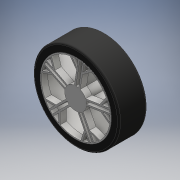
# Autodesk Inventor part: rueda
Saved by Autodesk Inventor 2016 (Build 200138000, 138)
## iProperties
Created: 2017-12-28
Part Number: rueda
Material: Genérico
Document SubType Name: Sheet Metal
Designer: David
Density: 1 g/cm^3
Sheet Metal Rule: Por defecto_mm
Appearance: Valor por defecto
Author: David
Autodesk Inventor part; units mm, degrees
ref_plane "YZ Plane" through (0, 0, 0) normal (1, 0, 0) x (0, 1, 0)
ref_plane "XZ Plane" through (0, 0, 0) normal (0, 1, 0) x (-1, 0, 0)
ref_plane "XY Plane" through (0, 0, 0) normal (0, 0, 1) x (1, 0, 0)
sketch "Boceto1" plane through (0, 0, 0) normal (0, 1, 0) x (-1, 0, 0)
  line L0 (0, 0) -> (10.7734, 0) construction
  line L1 (0, 0) -> (5.8764, 0) construction
  line L2 (0, 0) -> (5.8764, 0) construction
  line L3 (2.6962, -2.1086) -> (2.8923, -2.3046)
  line L4 (2.0927, -2.7086) -> (2.3729, -2.9905)
  line L5 (2.3729, -2.9905) -> (7.2915, -7.9381)
  line L6 (1.6666, -2.9897) -> (4.8298, -6.1715)
  line L7 (4.8298, -6.1715) -> (4.8298, -9.636)
  line L8 (5.3412, -9.3623) -> (5.3412, -6.6658)
  line L9 (5.3412, -6.6658) -> (6.9255, -8.2594)
  line L10 (2.6945, -2.1068) -> (2.9764, -2.387)
  line L11 (2.9764, -2.387) -> (7.924, -7.3056)
  line L12 (2.9755, -1.6808) -> (6.1574, -4.8439)
  line L13 (6.1574, -4.8439) -> (9.6219, -4.8439)
  line L14 (9.3481, -5.3553) -> (6.6517, -5.3553)
  line L15 (6.6517, -5.3553) -> (8.2453, -6.9396)
  line L16 (7.9237, -7.3054) -> (7.9246, -7.3062)
  line L17 (8.2447, -6.939) -> (8.2465, -6.9408)
  line L18 (9.3479, -5.3553) -> (9.3542, -5.3553)
  line L19 (9.6216, -4.8439) -> (9.6289, -4.8439)
  line L20 (7.1487, 4.6712) -> (9.1479, 5.6973)
  line L21 (7.982, 7.2357) -> (7.1487, 4.6712)
  line L22 (6.5096, 4.3592) -> (7.5802, 7.6541)
  line L23 (2.518, 2.3105) -> (6.5096, 4.3592)
  line L24 (3.19, 2.0931) -> (9.3967, 5.2786)
  line L25 (3.5774, 1.3327) -> (9.8028, 4.4816)
  line L26 (2.8363, 1.9116) -> (3.19, 2.0931)
  line L27 (3.2227, 1.1532) -> (3.5774, 1.3327)
  line L28 (3.3584, 0.6612) -> (7.362, 2.6863)
  line L29 (7.9901, 3.0199) -> (9.9953, 4.0342)
  line L30 (10.5546, 2.1867) -> (7.9901, 3.0199)
  line L31 (7.362, 2.6863) -> (10.6569, 1.6157)
  line L32 (-2.2335, 8.2423) -> (-2.5916, 10.4607)
  line L33 (-4.415, 9.8272) -> (-2.2335, 8.2423)
  line L34 (-2.1342, 7.538) -> (-4.9371, 9.5744)
  line L35 (-1.4193, 3.1088) -> (-2.1342, 7.538)
  line L36 (-1.0049, 3.6806) -> (-2.1165, 10.568)
  line L37 (-0.162, 3.8141) -> (-1.233, 10.7079)
  line L38 (-0.9415, 3.2882) -> (-1.0049, 3.6806)
  line L39 (-0.1009, 3.4214) -> (-0.162, 3.8141)
  line L40 (0.409, 3.3983) -> (-0.2799, 7.8318)
  line L41 (-0.4031, 8.5322) -> (-0.7481, 10.7527)
  line L42 (1.1819, 10.7137) -> (-0.4031, 8.5322)
  line L43 (-0.2799, 7.8318) -> (1.7565, 10.6346)
  line L44 (-8.5291, 0.4228) -> (-10.7496, 0.7678)
  line L45 (-10.7106, -1.1621) -> (-8.5291, 0.4228)
  line L46 (-7.8286, 0.2996) -> (-10.6315, -1.7368)
  line L47 (-3.3952, -0.3892) -> (-7.8286, 0.2996)
  line L48 (-3.811, 0.1817) -> (-10.7048, 1.2528)
  line L49 (-3.6775, 1.0246) -> (-10.5649, 2.1363)
  line L50 (-3.4182, 0.1207) -> (-3.811, 0.1817)
  line L51 (-3.2851, 0.9613) -> (-3.6775, 1.0246)
  line L52 (-3.1056, 1.4391) -> (-7.5349, 2.154)
  line L53 (-8.2392, 2.2533) -> (-10.4576, 2.6113)
  line L54 (-9.8241, 4.4347) -> (-8.2392, 2.2533)
  line L55 (-7.5349, 2.154) -> (-9.5713, 4.9568)
  line L56 (-3.0378, -7.981) -> (-4.052, -9.9862)
  line L57 (-2.2045, -10.5455) -> (-3.0378, -7.981)
  line L58 (-2.7041, -7.3529) -> (-1.6335, -10.6478)
  line L59 (-0.679, -3.3493) -> (-2.7041, -7.3529)
  line L60 (-1.3505, -3.5683) -> (-4.4994, -9.7937)
  line L61 (-2.1109, -3.1809) -> (-5.2964, -9.3877)
  line L62 (-1.1711, -3.2136) -> (-1.3505, -3.5683)
  line L63 (-1.9294, -2.8273) -> (-2.1109, -3.1809)
  line L64 (-2.3283, -2.5089) -> (-4.377, -6.5005)
  line L65 (-4.689, -7.1396) -> (-5.7151, -9.1388)
  line L66 (-7.2535, -7.9729) -> (-4.689, -7.1396)
  line L67 (-4.377, -6.5005) -> (-7.6719, -7.5711)
  arc A0 (3.2227, 1.1532) -> (2.8386, 1.9127) centre (0, 0) ccw
  arc A1 (2.9795, -1.6847) -> (3.3584, 0.6612) centre (0, 0) ccw
  arc A2 (2.0927, -2.7086) -> (2.6962, -2.1086) centre (0, 0) ccw
  arc A3 (-0.6815, -3.3543) -> (1.6666, -2.9897) centre (0, 0) ccw
  arc A4 (2.523, 2.3131) -> (0.409, 3.3983) centre (0, 0) ccw
  arc A5 (-0.1009, 3.4214) -> (-0.9419, 3.2907) centre (0, 0) ccw
  arc A6 (-1.4202, 3.1143) -> (-3.1056, 1.4391) centre (0, 0) ccw
  arc A7 (-3.2851, 0.9613) -> (-3.4207, 0.1211) centre (0, 0) ccw
  arc A8 (-3.4007, -0.3883) -> (-2.3283, -2.5089) centre (0, 0) ccw
  arc A9 (-1.9294, -2.8273) -> (-1.1722, -3.2159) centre (0, 0) ccw
  line L68 (-2.2052, -10.5433) -> (-2.2028, -10.5512)
  line L69 (-1.6344, -10.645) -> (-1.6314, -10.6545)
  line L70 (-4.0517, -9.9854) -> (-4.0528, -9.9877)
  line L71 (-4.4993, -9.7934) -> (-4.4998, -9.7945)
  line L72 (-10.6191, -1.7278) -> (-10.6372, -1.7409)
  line L73 (-10.7085, -1.1606) -> (-10.7155, -1.1657)
  line L74 (-10.748, 0.7676) -> (-10.7513, 0.7681)
  line L75 (-10.702, 1.2524) -> (-10.7056, 1.2529)
  line L76 (-4.9362, 9.5738) -> (-4.9428, 9.5786)
  line L77 (-4.413, 9.8258) -> (-4.4199, 9.8308)
  line L78 (-2.5912, 10.4584) -> (-2.5918, 10.4624)
  line L79 (-2.1163, 10.567) -> (-2.1166, 10.5688)
  line L80 (7.5795, 7.652) -> (7.5824, 7.6608)
  line L81 (7.9813, 7.2335) -> (7.9838, 7.2415)
  line L82 (9.1453, 5.6959) -> (9.1494, 5.6981)
  line L83 (9.395, 5.2777) -> (9.3975, 5.279)
  circle A10 centre (0, 0) radius 11.15
  arc A11 (9.1494, 5.6981) -> (7.9838, 7.2415) centre (0, 0) ccw
  arc A12 (9.8028, 4.4816) -> (9.3975, 5.279) centre (0, 0) ccw
  arc A13 (10.5546, 2.1867) -> (9.9953, 4.0342) centre (0, 0) ccw
  arc A14 (9.6289, -4.8439) -> (10.6569, 1.6157) centre (0, 0) ccw
  arc A15 (8.2465, -6.9408) -> (9.3542, -5.3553) centre (0, 0) ccw
  arc A16 (7.2915, -7.9381) -> (7.9246, -7.3062) centre (0, 0) ccw
  arc A17 (5.3412, -9.3623) -> (6.9255, -8.2594) centre (0, 0) ccw
  arc A18 (-5.2964, -9.3877) -> (-4.4998, -9.7945) centre (0, 0) ccw
  arc A19 (-4.0528, -9.9877) -> (-2.2028, -10.5512) centre (0, 0) ccw
  arc A20 (-1.6314, -10.6545) -> (4.8298, -9.636) centre (0, 0) ccw
  arc A21 (-7.2535, -7.9729) -> (-5.7151, -9.1388) centre (0, 0) ccw
  arc A22 (7.5824, 7.6608) -> (1.7565, 10.6346) centre (0, 0) ccw
  arc A23 (1.1819, 10.7137) -> (-0.7481, 10.7527) centre (0, 0) ccw
  arc A24 (-1.233, 10.7079) -> (-2.1166, 10.5688) centre (0, 0) ccw
  arc A25 (-2.5918, 10.4624) -> (-4.4199, 9.8308) centre (0, 0) ccw
  arc A26 (-4.9428, 9.5786) -> (-9.5713, 4.9568) centre (0, 0) ccw
  arc A27 (-9.8241, 4.4347) -> (-10.4576, 2.6113) centre (0, 0) ccw
  arc A28 (-10.5649, 2.1363) -> (-10.7056, 1.2529) centre (0, 0) ccw
  arc A29 (-10.7513, 0.7681) -> (-10.7155, -1.1657) centre (0, 0) ccw
  arc A30 (-10.6372, -1.7409) -> (-7.6719, -7.5711) centre (0, 0) ccw
  point P0 (9.1472, 5.6969)
  point P1 (7.9819, 7.2355)
  point P2 (7.5801, 7.6539)
  point P3 (9.3964, 5.2784)
  point P4 (-2.5914, 10.4599)
  point P5 (-4.4148, 9.8271)
  point P6 (-4.9369, 9.5743)
  point P7 (-2.1164, 10.5676)
  point P8 (-10.7487, 0.7677)
  point P9 (-10.7104, -1.162)
  point P10 (-10.6313, -1.7366)
  point P11 (-10.7044, 1.2527)
  point P12 (-2.2046, -10.5453)
  point P13 (-1.6336, -10.6476)
  dimension "d18" = 360
  constraints: 168 end point, 61 point on circle, 55 point on line, 31 centre point, 5 horizontal, 3 coincident, 2 parallel, 2 vertical, 1 collinear, 171 other
extrude "Extrusión1" add sketch "Boceto1" along normal blind 2
sketch "Boceto7" plane through (0, 2, 0) normal (0, 1, 0) x (1, 0, 0)
  circle A0 centre (0, 0) radius 11.15
  circle A1 centre (0, 0) radius 13.5
  dimension "d31" = 27
  constraints: 2 centre point, 2 coincident
  measures "d31" diameter of A1
extrude "Extrusión5" add sketch "Boceto7" along normal blind 7
sketch "Boceto8" plane through (0, 2, 0) normal (0, -1, 0) x (1, 0, 0)
  circle A0 centre (0, 0) radius 11.15
  circle A1 centre (0, 0) radius 13.5
  dimension "d34" = 27
  constraints: 2 centre point, 2 coincident
  measures "d34" diameter of A1
extrude "Extrusión6" add sketch "Boceto8" along normal blind 1.9
sketch "Boceto9" plane through (0, 2, 0) normal (0, 1, 0) x (1, 0, 0)
  line L0 (3.4207, -0.1211) -> (10.7056, -1.2529) projected
  line L1 (0.2361, -0.0276) -> (10.7056, -1.2529)
  line L2 (10.7056, -1.2529) -> (10.7487, -0.9756)
  line L3 (10.7487, -0.9756) -> (0.1231, 0.268)
  line L4 (4.4998, 9.7945) -> (1.1722, 3.2159) projected
  arc A0 (4.0528, 9.9877) -> (2.2028, 10.5512) centre (0, 0) ccw projected
  line L5 (4.4998, 9.7945) -> (0.1231, 0.268)
  line L6 (4.4998, 9.7945) -> (4.2815, 9.8919)
  line L7 (4.2815, 9.8919) -> (-0.1767, 0.1629)
  line L8 (-7.9246, 7.3062) -> (-2.6962, 2.1086) projected
  line L9 (-0.1767, 0.1629) -> (-7.9246, 7.3062)
  arc A1 (-7.2915, 7.9381) -> (-7.9246, 7.3062) centre (0, 0) ccw projected
  line L10 (-7.9246, 7.3062) -> (-8.069, 7.1497)
  line L11 (-8.069, 7.1497) -> (-0.652, 0.0763)
  line L12 (-2.8386, -1.9127) -> (-9.3975, -5.279) projected
  line L13 (-0.3599, -0.2022) -> (-9.3975, -5.279)
  line L14 (-9.3975, -5.279) -> (-9.2863, -5.4722)
  line L15 (-9.2863, -5.4722) -> (0, -0.2897)
  line L16 (0.9419, -3.2907) -> (2.1166, -10.5688) projected
  line L17 (0.0508, -0.2536) -> (2.1166, -10.5688)
  line L18 (2.1166, -10.5688) -> (2.34, -10.5328)
  line L19 (2.34, -10.5328) -> (0.2361, -0.0276)
  line L20 (-0.652, 0.0763) -> (-0.3599, -0.2022)
  line L21 (0, -0.2897) -> (0.0508, -0.2536)
  constraints: 34 end point, 2 parallel, 2 perpendicular, 1 tangent
extrude "Extrusión7" add sketch "Boceto9" along normal blind 6.5
sketch "Boceto10" plane through (0, 8.5, 0) normal (0, 1, 0) x (1, 0, 0)
  circle A0 centre (0, 0) radius 2.5
  dimension "d39" = 5
  constraints: 1 centre point, 1 coincident
  measures "d39" diameter of A0
extrude "Extrusión8" add sketch "Boceto10" against normal blind 6.5
fillet "Empalme1" radius 0.5 1 edges at (-13.5, 0.1, 0)
fillet "Empalme2" radius 0.5 1 edges at (-13.5, 9, 0)
equation "\"Radio_pliegue\" = Grosor"
equation "\"Anchura_desahogo_plegado\" = Grosor"
equation "\"Profundidad_desahogo_plegado\" = 0.5 * Grosor"
equation "\"Tamaño_destalonado\" = 4 * Grosor"
equation "\"Remanente_mínimo\" = 2 * Grosor"
equation "\"Radiodetransición\" = Radio_pliegue"
equation "\"Tamaño_de_radio_de_Jacobi\" = Radio_pliegue"
equation "\"TamañoSeparación\" = Grosor"
equation "\"Grosor\" = 0.5"
